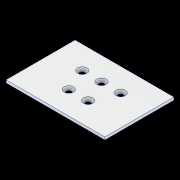
# Autodesk Inventor part: MetalFrontWedge
Saved by Autodesk Inventor 2021 (Build 250183000, 183)
## iProperties
Created: 2020-10-21
Part Number: MetalFrontWedge
Material: Aluminum 6061
Document SubType Name: Sheet Metal
Designer: Esketitttttt
Mass: 7.71591 g
Surface Area: 39.2202 cm^2
Volume: 2.85775 cm^3
Density: 2.7 g/cm^3
Sheet Metal Rule: Default
Appearance: Aluminum - Flat
Author: Esketitttttt
Autodesk Inventor part; units mm, degrees
ref_plane "YZ Plane" through (0, 0, 0) normal (1, 0, 0) x (0, 1, 0)
ref_plane "XZ Plane" through (0, 0, 0) normal (0, 1, 0) x (-1, 0, 0)
ref_plane "XY Plane" through (0, 0, 0) normal (0, 0, 1) x (1, 0, 0)
sketch "Sketch1" plane through (0, 0, 0) normal (0, 1, 0) x (-1, 0, 0)
  circle A0 centre (11.26, 13.4426) radius 1.016
  circle A1 centre (28.15, 26.8853) radius 1.016
  circle A2 centre (16.89, 26.8853) radius 1.016
  circle A3 centre (22.52, 13.4426) radius 1.016
  circle A4 centre (33.78, 13.4426) radius 1.016
  line L0 (0, 0) -> (0, 40.3279)
  line L1 (45.04, 0) -> (0, 0)
  line L2 (45.04, 40.3279) -> (45.04, 0)
  line L3 (0, 40.3279) -> (45.04, 40.3279)
  line L4 (0, 40.3279) -> (-6.35, 40.3279)
  line L5 (-6.35, 40.3279) -> (-6.35, 0)
  line L6 (-6.35, 0) -> (0, 0)
  line L7 (0, 0) -> (0, 40.3279)
  line L8 (45.04, 40.3279) -> (51.39, 40.3279)
  line L9 (51.39, 40.3279) -> (51.39, 0)
  line L10 (51.39, 0) -> (45.04, 0)
  line L11 (45.04, 0) -> (45.04, 40.3279)
  point P0 (-38.1, 53.4116)
  dimension "d1" = 6.35
  dimension "d2" = 6.35
  measures "d1" distance of L6.end L5.end
  measures "d2" distance of L9.end L10.end
extrude "Plate1" add sketch "Sketch1" along normal blind 1.5875
sketch "Sketch2" plane through (0, 1.5875, 0) normal (0, 1, 0) x (1, 0, 0)
  circle A0 centre (-33.78, -13.4426) radius 1.016 projected
  circle A1 centre (-22.52, -13.4426) radius 1.016 projected
  circle A2 centre (-16.89, -26.8853) radius 1.016 projected
  circle A3 centre (-11.26, -13.4426) radius 1.016 projected
  circle A4 centre (-33.78, -13.4426) radius 1.016 projected
  circle A5 centre (-22.52, -13.4426) radius 1.016 projected
  circle A6 centre (-16.89, -26.8853) radius 1.016 projected
  circle A7 centre (-28.15, -26.8853) radius 1.016 projected
  circle A8 centre (-11.26, -13.4426) radius 1.016 projected
  line L0 (6.35, -40.3279) -> (-51.39, -40.3279) projected
  line L1 (6.35, 0) -> (6.35, -40.3279) projected
  line L2 (-51.39, 0) -> (6.35, 0) projected
  line L3 (-51.39, -40.3279) -> (-51.39, 0) projected
hole "Hole2" at (-28.15, 1.5875, 26.8853) at (-33.78, 1.5875, 13.4426) at (-22.52, 1.5875, 13.4426) at (-11.26, 1.5875, 13.4426) at (-16.89, 1.5875, 26.8853) direction (0, -1, 0) diameter 2.8448 end through all countersink diameter 5.461 countersink angle 82
equation "\"d15\" = Thickness"
equation "\"d0\" = Thickness"
equation "\"BendRadius\" = Thickness"
equation "\"BendReliefWidth\" = Thickness"
equation "\"BendReliefDepth\" = 0.5 * Thickness"
equation "\"CornerReliefSize\" = 4 * Thickness"
equation "\"MinimumRemnant\" = 2 * Thickness"
equation "\"TransitionRadius\" = BendRadius"
equation "\"JacobiRadiusSize\" = BendRadius"
equation "\"GapSize\" = Thickness"
equation "\"Thickness\" = 1.5875"
body "Solid1"
